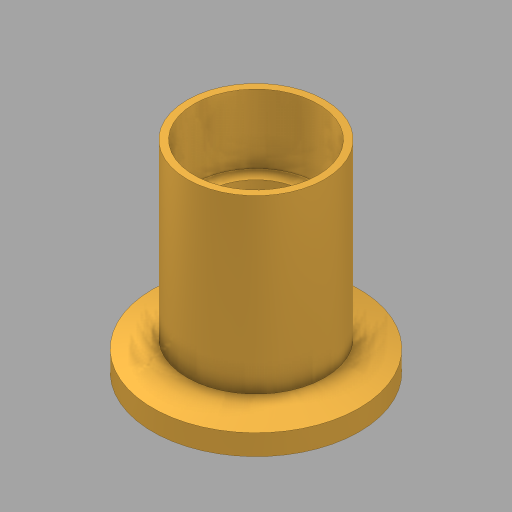
# Autodesk Inventor part: EpoxyFitThroughKF16
Saved by Autodesk Inventor 2024 (Build 280153020, 153B)
## iProperties
Created: 2023-10-02
Part Number: EpoxyFitThroughKF16
Material: Brass, Soft Yellow
Document SubType Name: Modeling
Designer: schanen
Density: 8.47 g/cm^3
Appearance: Brass - Satin
Author: schanen
Autodesk Inventor part; units mm, degrees
ref_plane "YZ Plane" through (0, 0, 0) normal (1, 0, 0) x (0, 1, 0)
ref_plane "XZ Plane" through (0, 0, 0) normal (0, 1, 0) x (-1, 0, 0)
ref_plane "XY Plane" through (0, 0, 0) normal (0, 0, 1) x (1, 0, 0)
sketch "Sketch1" plane through (0, 0, 0) normal (0, 0, 1) x (1, 0, 0)
  line L0 (-15, 0) -> (-15, 3)
  line L1 (-15, 3) -> (-10, 4.3397)
  line L2 (-10, 4.3397) -> (-10, 19.3397)
  line L3 (-7, 19.3397) -> (-7, 2.5)
  line L4 (-7, 2.5) -> (-8.75, 2.5)
  line L5 (-8.75, 2.5) -> (-8.75, 0)
  line L6 (-8.75, 0) -> (-15, 0)
  line L7 (-10, 19.3397) -> (-10, 29.3397)
  line L8 (-10, 29.3397) -> (-9, 29.3397)
  line L9 (-9, 29.3397) -> (-9, 19.3397)
  line L10 (-9, 19.3397) -> (-7, 19.3397)
  line L11 (0, -5.8679) -> (0, 35.2077) projected
  point P0 (0, 0)
  dimension "d0" = 8.75
  dimension "d1" = 15
  dimension "d2" = 3
  dimension "d4" = 15
  dimension "d6" = 2.5
  dimension "d7" = 10
  dimension "d8" = 7
  dimension "d9" = 15
  dimension "d10" = 10
  dimension "d11" = 1
  constraints: 22 end point, 5 perpendicular, 3 vertical, 2 horizontal alignment, 1 horizontal, 1 parallel
  measures "d0" distance from line of point (0, 0) L5
  measures "d1" distance from line of point (0, 0) L0
  measures "d2" distance of L0.start L0.end
  measures "d4" angle of L6 L1
  measures "d6" distance of L4.end L5.end
  measures "d7" distance from line of point (0, 0) L2
  measures "d8" distance from line of point (0, 0) L3
  measures "d9" distance of L1.end L2.end
  measures "d10" distance of L2.end L7.end
  measures "d11" distance between parallel lines of L9 L7
revolve "Revolution1" add sketch "Sketch1" angle 360 about axis through (0, -10, 0) along (0, 1, 0)
body "Solid1"
